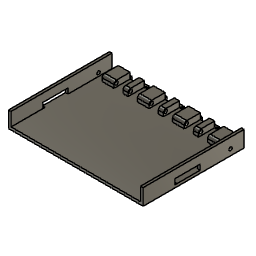
NEW+Key+Housing (Autodesk Fusion 360 design; units mm, degrees)
Autodesk Fusion 360 part; units mm, degrees
note: some values were not read from the file. Set by a fixed rule: which sketch regions a step uses.
sketch "Base" plane through (0, 0, 0) normal (0, 0, 1) x (1, 0, 0)
  line L0 (0, 0) -> (101.6, 0)
  line L1 (101.6, 0) -> (101.6, 76.2)
  line L2 (0, 0) -> (0, 76.2)
  line L3 (0, 76.2) -> (0, 78.74)
  line L4 (0, 78.74) -> (101.6, 78.74)
  line L5 (101.6, 78.74) -> (101.6, 76.2)
  dimension "d1" = 101.6
  dimension "d2" = 76.2
  dimension "d3" = 76.2
  dimension "d24" = 2.54
  dimension "d25" = 101.6
  constraint coincident L0.start L2.start
  constraint horizontal L0
  constraint perpendicular L0 L1
  constraint perpendicular L0 L2
  constraint perpendicular L3 L4
  constraint vertical L5
  measures "d1" distance of L0.start L0.end
  measures "d2" distance of L0.end L1.end
  measures "d3" distance of L0.start L2.end
  measures "d24" distance of L2.end L3.end
  measures "d25" distance of L3.end L4.end
extrude "Extrude1" add sketch "Base" along normal blind 2.032
sketch "back fins" plane through (0, 0, 2.032) normal (0, 0, 1) x (-1, 0, 0)
  line L0 (0, 0) -> (-101.6, 0)
  line L1 (-101.6, 0) -> (-101.6, -76.2)
  line L2 (-101.6, -76.2) -> (-101.6, -78.74)
  line L3 (0, -78.74) -> (0, 0)
  line L4 (0, -78.74) -> (0, -76.2)
  line L5 (0, -76.2) -> (-5.969, -76.2)
  line L6 (-16.129, -76.2) -> (-5.969, -76.2)
  line L7 (0, -78.74) -> (0, -76.2)
  line L8 (-5.969, -76.2) -> (0, -76.2)
  line L9 (-16.129, -76.2) -> (-21.209, -76.2)
  line L10 (-27.432, -76.2) -> (-21.209, -76.2)
  line L11 (-27.432, -76.2) -> (-32.512, -76.2)
  line L12 (-32.512, -76.2) -> (-42.672, -76.2)
  line L13 (-42.672, -76.2) -> (-47.752, -76.2)
  line L14 (-53.975, -76.2) -> (-59.055, -76.2)
  line L15 (-69.215, -76.2) -> (-59.055, -76.2)
  line L16 (-47.752, -76.2) -> (-53.975, -76.2)
  line L17 (-69.215, -76.2) -> (-74.295, -76.2)
  line L18 (-101.6, -78.74) -> (-101.6, -76.2)
  line L19 (-11.049, -76.2) -> (-11.049, -78.74)
  line L20 (-24.3205, -76.2) -> (-24.3205, -78.74)
  line L21 (-37.592, -76.2) -> (-37.592, -78.74)
  line L22 (-50.8635, -76.2) -> (-50.8635, -78.74)
  line L23 (-64.135, -76.2) -> (-64.135, -78.74)
  line L24 (-77.4065, -76.2) -> (-77.4065, -78.74)
  line L25 (-90.678, -76.2) -> (-90.678, -78.74)
  line L26 (-11.049, -78.74) -> (-7.6835, -78.74)
  line L27 (-11.049, -78.74) -> (-14.4145, -78.74)
  line L28 (-24.3205, -78.74) -> (-20.955, -78.74)
  line L29 (-24.3205, -78.74) -> (-27.686, -78.74)
  line L30 (-37.592, -78.74) -> (-40.9575, -78.74)
  line L31 (-50.8635, -78.74) -> (-47.498, -78.74)
  line L32 (-50.8635, -78.74) -> (-54.229, -78.74)
  line L33 (-64.135, -78.74) -> (-60.7695, -78.74)
  line L34 (-64.135, -78.74) -> (-67.5005, -78.74)
  line L35 (-77.4065, -78.74) -> (-80.772, -78.74)
  line L36 (-90.678, -78.74) -> (-87.3125, -78.74)
  line L37 (-90.678, -78.74) -> (-94.0435, -78.74)
  line L38 (-37.592, -78.74) -> (-34.2265, -78.74)
  line L39 (-74.295, -76.2) -> (-101.6, -76.2)
  line L40 (-7.6835, -78.74) -> (-7.6835, -77.47)
  line L41 (-7.6835, -77.47) -> (-8.9535, -77.47)
  line L42 (-8.9535, -77.47) -> (-8.9535, -76.2)
  line L43 (-14.4145, -78.74) -> (-14.4145, -77.47)
  line L44 (-14.4145, -77.47) -> (-13.1445, -77.47)
  line L45 (-13.1445, -77.47) -> (-13.1445, -76.2)
  line L46 (-20.955, -78.74) -> (-20.955, -77.47)
  line L47 (-20.955, -77.47) -> (-22.225, -77.47)
  line L48 (-22.225, -77.47) -> (-22.225, -76.2)
  line L49 (-27.686, -78.74) -> (-27.686, -77.47)
  line L50 (-27.686, -77.47) -> (-26.416, -77.47)
  line L51 (-26.416, -77.47) -> (-26.416, -76.2)
  line L52 (-34.2265, -78.74) -> (-34.2265, -77.47)
  line L53 (-34.2265, -77.47) -> (-35.4965, -77.47)
  line L54 (-35.4965, -77.47) -> (-35.4965, -76.2)
  line L55 (-40.9575, -78.74) -> (-40.9575, -77.47)
  line L56 (-40.9575, -77.47) -> (-39.6875, -77.47)
  line L57 (-39.6875, -77.47) -> (-39.6875, -76.2)
  line L58 (-47.498, -78.74) -> (-47.498, -77.47)
  line L59 (-47.498, -77.47) -> (-48.768, -77.47)
  line L60 (-48.768, -77.47) -> (-48.768, -76.2)
  line L61 (-54.229, -78.74) -> (-54.229, -77.47)
  line L62 (-54.229, -77.47) -> (-52.959, -77.47)
  line L63 (-52.959, -77.47) -> (-52.959, -76.2)
  line L64 (-60.7695, -78.74) -> (-60.7695, -77.47)
  line L65 (-67.5005, -78.74) -> (-67.5005, -77.47)
  line L66 (-60.7695, -77.47) -> (-62.0395, -77.47)
  line L67 (-67.5005, -77.47) -> (-66.2305, -77.47)
  line L68 (-62.0395, -77.47) -> (-62.0395, -76.2)
  line L69 (-66.2305, -77.47) -> (-66.2305, -76.2)
  line L70 (-80.772, -78.74) -> (-80.772, -77.47)
  line L71 (-22.4155, -76.2) -> (-26.2255, -76.2)
  line L72 (-80.772, -77.47) -> (-79.502, -77.47)
  line L73 (-79.502, -77.47) -> (-79.502, -76.2)
  line L74 (-77.4065, -78.74) -> (-74.0283, -78.74)
  line L75 (-74.0283, -78.74) -> (-74.0283, -77.47)
  line L76 (-74.0283, -77.47) -> (-75.2983, -77.47)
  line L77 (-75.2983, -77.47) -> (-75.2983, -76.2)
  line L78 (-87.3125, -78.74) -> (-87.3125, -77.47)
  line L79 (-87.3125, -77.47) -> (-88.5825, -77.47)
  line L80 (-88.5825, -77.47) -> (-88.5825, -76.2)
  line L81 (-94.0435, -78.74) -> (-94.0435, -77.47)
  line L82 (-94.0435, -77.47) -> (-92.7735, -77.47)
  line L83 (-92.7735, -77.47) -> (-92.7735, -76.2)
  line L84 (0, -76.2) -> (0, -78.74)
  line L85 (0, -78.74) -> (-7.6835, -78.74)
  line L86 (-14.4145, -78.74) -> (-20.955, -78.74)
  line L87 (-27.686, -78.74) -> (-34.2265, -78.74)
  line L88 (-40.9575, -78.74) -> (-47.498, -78.74)
  line L89 (-54.229, -78.74) -> (-60.7695, -78.74)
  line L90 (-67.5005, -78.74) -> (-74.0283, -78.74)
  line L91 (-80.772, -78.74) -> (-87.3125, -78.74)
  line L92 (-94.0435, -78.74) -> (-101.6, -78.74)
  dimension "d27" = 5.969
  dimension "d118" = 3.3655
  dimension "d119" = 3.3655
  dimension "d120" = 3.3655
  dimension "d121" = 3.3655
  dimension "d123" = 3.3655
  dimension "d124" = 3.3655
  dimension "d125" = 3.3655
  dimension "d126" = 3.3655
  dimension "d127" = 3.3655
  dimension "d129" = 3.3655
  dimension "d130" = 3.3655
  dimension "d131" = 3.3655
  dimension "d132" = 3.3655
  dimension "d133" = 1.27
  dimension "d134" = 1.27
  dimension "d135" = 1.27
  dimension "d136" = 1.27
  dimension "d137" = 1.27
  dimension "d138" = 1.27
  dimension "d139" = 1.27
  dimension "d140" = 1.27
  dimension "d141" = 1.27
  dimension "d142" = 1.27
  dimension "d143" = 1.27
  dimension "d144" = 1.27
  dimension "d145" = 1.27
  dimension "d146" = 1.27
  dimension "d147" = 1.27
  dimension "d148" = 1.27
  dimension "d149" = 1.27
  dimension "d150" = 1.27
  dimension "d151" = 1.27
  dimension "d152" = 1.27
  dimension "d153" = 1.27
  dimension "d156" = 1.27
  dimension "d157" = 3.81
  dimension "d159" = 1.27
  dimension "d161" = 3.3782
  dimension "d162" = 1.27
  dimension "d163" = 1.27
  dimension "d164" = 1.27
  dimension "d165" = 1.27
  dimension "d166" = 1.27
  dimension "d167" = 1.27
  constraint coincident L3.start L4.start
  constraint coincident L3 L4.end
  constraint perpendicular L4 L5
  constraint coincident L2.end L18.start
  constraint coincident L1.end L2.start
  constraint midpoint L6 L19.start
  constraint midpoint L10 L20.start
  constraint midpoint L12 L21.start
  constraint midpoint L16 L22.start
  constraint midpoint L15 L23.start
  constraint perpendicular L19 L26
  constraint perpendicular L19 L27
  constraint perpendicular L20 L28
  constraint perpendicular L20 L29
  constraint perpendicular L21 L30
  constraint perpendicular L22 L31
  constraint perpendicular L22 L32
  constraint perpendicular L23 L33
  constraint perpendicular L23 L34
  constraint perpendicular L24 L35
  constraint perpendicular L25 L36
  constraint perpendicular L25 L37
  constraint perpendicular L21 L38
  constraint perpendicular L26 L40
  constraint perpendicular L40 L41
  constraint coincident L6 L42.end
  constraint perpendicular L6 L42
  constraint perpendicular L27 L43
  constraint perpendicular L43 L44
  constraint coincident L6 L45.end
  constraint perpendicular L6 L45
  constraint perpendicular L28 L46
  constraint perpendicular L46 L47
  constraint coincident L10 L48.end
  constraint perpendicular L10 L48
  constraint perpendicular L29 L49
  constraint perpendicular L49 L50
  constraint coincident L10 L51.end
  constraint perpendicular L10 L51
  constraint perpendicular L38 L52
  constraint perpendicular L52 L53
  constraint coincident L12 L54.end
  constraint perpendicular L12 L54
  constraint perpendicular L30 L55
  constraint perpendicular L55 L56
  constraint coincident L12 L57.end
  constraint perpendicular L12 L57
  constraint perpendicular L31 L58
  constraint perpendicular L58 L59
  constraint coincident L16 L60.end
  constraint perpendicular L16 L60
  constraint perpendicular L32 L61
  constraint perpendicular L61 L62
  constraint perpendicular L16 L63
  constraint perpendicular L33 L64
  constraint perpendicular L34 L65
  constraint perpendicular L64 L66
  constraint perpendicular L65 L67
  constraint coincident L15 L68.end
  constraint perpendicular L15 L68
  constraint coincident L15 L69.end
  constraint perpendicular L15 L69
  constraint perpendicular L35 L70
  constraint horizontal L71
  constraint perpendicular L70 L72
  constraint coincident L39 L73.end
  constraint perpendicular L39 L73
  constraint perpendicular L24 L74
  constraint perpendicular L74 L75
  constraint perpendicular L75 L76
  constraint coincident L39 L77.end
  constraint perpendicular L39 L77
  constraint perpendicular L36 L78
  constraint perpendicular L78 L79
  constraint coincident L39 L80.end
  constraint perpendicular L39 L80
  constraint perpendicular L37 L81
  constraint perpendicular L81 L82
  constraint coincident L39 L83.end
  constraint perpendicular L39 L83
  constraint perpendicular L40 L85
  constraint perpendicular L46 L86
  constraint perpendicular L52 L87
  constraint perpendicular L58 L88
  constraint perpendicular L64 L89
  constraint perpendicular L75 L90
  constraint perpendicular L78 L91
  constraint parallel L37 L92
  measures "d27" distance of L4.end L5.end
  measures "d118" distance of L19.end L26.end
  measures "d119" distance of L19.end L27.end
  measures "d120" distance of L20.end L28.end
  measures "d121" distance of L20.end L29.end
  measures "d123" distance of L21.end L30.end
  measures "d124" distance of L22.end L31.end
  measures "d125" distance of L22.end L32.end
  measures "d126" distance of L23.end L33.end
  measures "d127" distance of L23.end L34.end
  measures "d129" distance of L24.end L35.end
  measures "d130" distance of L25.end L36.end
  measures "d131" distance of L25.end L37.end
  measures "d132" distance of L21.end L38.end
  measures "d133" distance of L26.end L40.end
  measures "d134" distance of L40.end L41.end
  measures "d135" distance of L27.end L43.end
  measures "d136" distance of L43.end L44.end
  measures "d137" distance of L28.end L46.end
  measures "d138" distance of L46.end L47.end
  measures "d139" distance of L29.end L49.end
  measures "d140" distance of L49.end L50.end
  measures "d141" distance of L38.end L52.end
  measures "d142" distance of L52.end L53.end
  measures "d143" distance of L30.end L55.end
  measures "d144" distance of L55.end L56.end
  measures "d145" distance of L31.end L58.end
  measures "d146" distance of L58.end L59.end
  measures "d147" distance of L32.end L61.end
  measures "d148" distance of L61.end L62.end
  measures "d149" distance of L62.end L63.end
  measures "d150" distance of L33.end L64.end
  measures "d151" distance of L34.end L65.end
  measures "d152" distance of L64.end L66.end
  measures "d153" distance of L65.end L67.end
  measures "d156" distance of L35.end L70.end
  measures "d157" distance of L71.end L71.start
  measures "d159" distance of L70.end L72.end
  measures "d161" distance of L24.end L74.end
  measures "d162" distance of L74.end L75.end
  measures "d163" distance of L75.end L76.end
  measures "d164" distance of L36.end L78.end
  measures "d165" distance of L78.end L79.end
  measures "d166" distance of L37.end L81.end
  measures "d167" distance of L81.end L82.end
extrude "Extrude3" cut sketch "back fins" against normal blind 2.54 contours L3 L4 L5 L6 L7 L8 L40 L41 L42 L84 L85 | L2 L18 L39 L81 L82 L83 L92 | L39 L70 L72 L73 L78 L79 L80 L91 | L6 L9 L10 L43 L44 L45 L46 L47 L48 L86 | L15 L17 L39 L65 L67 L69 L75 L76 L77 L90 | L10 L11 L12 L49 L50 L51 L52 L53 L54 L87 | L12 L13 L16 L55 L56 L57 L58 L59 L60 L88 | L14 L15 L16 L61 L62 L63 L64 L66 L68 L89
sketch "axel fins" plane through (0, 0, 2.032) normal (0, 0, 1) x (-1, 0, 0)
  line L0 (-27.686, -78.74) -> (-20.955, -78.74)
  line L1 (-11.049, -78.74) -> (-11.049, -77.724)
  line L2 (-24.3205, -78.74) -> (-24.3205, -77.724)
  line L3 (-37.592, -78.74) -> (-37.592, -77.724)
  line L4 (-50.8635, -78.74) -> (-50.8635, -77.978)
  line L5 (-64.135, -78.74) -> (-64.135, -77.978)
  line L6 (-77.4065, -78.74) -> (-77.4065, -77.724)
  line L7 (-90.678, -78.74) -> (-90.678, -77.978)
  line L8 (-6.604, -76.2) -> (-15.494, -76.2)
  line L9 (-15.494, -76.2) -> (-15.494, -66.04)
  line L10 (-6.604, -66.04) -> (-6.604, -76.2)
  line L11 (-11.049, -76.2) -> (-11.049, -66.04)
  line L12 (-33.147, -76.2) -> (-42.037, -76.2)
  line L13 (-33.147, -60.96) -> (-33.147, -76.2)
  line L14 (-37.592, -76.2) -> (-37.592, -60.96)
  line L15 (-42.037, -60.96) -> (-33.147, -60.96)
  line L16 (-42.037, -76.2) -> (-42.037, -60.96)
  line L17 (-59.69, -76.2) -> (-68.58, -76.2)
  line L18 (-59.69, -60.96) -> (-59.69, -76.2)
  line L19 (-64.135, -76.2) -> (-64.135, -60.96)
  line L20 (-68.58, -60.96) -> (-59.69, -60.96)
  line L21 (-68.58, -76.2) -> (-68.58, -60.96)
  line L22 (-86.233, -76.2) -> (-95.123, -76.2)
  line L23 (-86.233, -60.96) -> (-86.233, -76.2)
  line L24 (-90.678, -76.2) -> (-90.678, -60.96)
  line L25 (-95.123, -60.96) -> (-86.233, -60.96)
  line L26 (-95.123, -76.2) -> (-95.123, -60.96)
  line L27 (-22.4155, -76.2) -> (-26.2255, -76.2)
  line L28 (-26.2255, -76.2) -> (-26.2255, -60.96)
  line L29 (-26.2255, -60.96) -> (-22.4155, -60.96)
  line L30 (-22.4155, -60.96) -> (-22.4155, -76.2)
  line L31 (-24.3205, -76.2) -> (-24.3205, -60.96)
  line L32 (-6.604, -76.2) -> (-15.494, -76.2)
  line L33 (-6.604, -66.04) -> (-6.604, -76.2)
  line L34 (-11.049, -76.2) -> (-11.049, -66.04)
  line L35 (-15.494, -76.2) -> (-15.494, -66.04)
  line L36 (-6.604, -76.2) -> (-15.494, -76.2)
  line L37 (-6.604, -60.96) -> (-6.604, -76.2)
  line L38 (-11.049, -76.2) -> (-11.049, -60.96)
  line L39 (-15.494, -60.96) -> (-6.604, -60.96)
  line L40 (-15.494, -76.2) -> (-15.494, -60.96)
  line L41 (-48.9585, -76.2) -> (-52.7685, -76.2)
  line L42 (-48.9585, -60.96) -> (-48.9585, -76.2)
  line L43 (-50.8635, -76.2) -> (-50.8635, -60.96)
  line L44 (-52.7685, -76.2) -> (-52.7685, -60.96)
  line L45 (-52.7685, -60.96) -> (-48.9585, -60.96)
  line L46 (-75.5015, -76.2) -> (-79.3115, -76.2)
  line L47 (-75.5015, -60.96) -> (-75.5015, -76.2)
  line L48 (-77.4065, -76.2) -> (-77.4065, -60.96)
  line L49 (-79.3115, -76.2) -> (-79.3115, -60.96)
  line L50 (-79.3115, -60.96) -> (-75.5015, -60.96)
  line L51 (-74.0283, -78.74) -> (-74.0283, -77.47)
  line L52 (-74.0283, -77.47) -> (-75.2983, -77.47)
  line L53 (-75.2983, -77.47) -> (-75.2983, -76.2)
  line L54 (-101.6, -76.2) -> (-92.7735, -76.2)
  line L55 (-7.6835, -78.74) -> (-7.6835, -77.47)
  line L56 (-7.6835, -77.47) -> (-8.9535, -77.47)
  line L57 (-8.9535, -77.47) -> (-8.9535, -76.2)
  line L58 (-21.209, -76.2) -> (-13.1445, -76.2)
  line L59 (-13.1445, -76.2) -> (-13.1445, -77.47)
  line L60 (-13.1445, -77.47) -> (-14.4145, -77.47)
  line L61 (-14.4145, -77.47) -> (-14.4145, -78.74)
  line L62 (-67.5005, -77.47) -> (-67.5005, -78.74)
  line L63 (-67.5005, -78.74) -> (-60.7695, -78.74)
  line L64 (-60.7695, -78.74) -> (-60.7695, -77.47)
  line L65 (-60.7695, -77.47) -> (-62.0395, -77.47)
  line L66 (-62.0395, -77.47) -> (-62.0395, -76.2)
  line L67 (-62.0395, -76.2) -> (-59.055, -76.2)
  line L68 (-66.2305, -76.2) -> (-66.2305, -77.47)
  line L69 (-66.2305, -77.47) -> (-67.5005, -77.47)
  line L70 (-54.229, -77.47) -> (-54.229, -78.74)
  line L71 (-54.229, -78.74) -> (-47.498, -78.74)
  line L72 (-47.498, -78.74) -> (-47.498, -77.47)
  line L73 (-47.498, -77.47) -> (-48.768, -77.47)
  line L74 (-48.768, -77.47) -> (-48.768, -76.2)
  line L75 (-59.055, -76.2) -> (-52.959, -76.2)
  line L76 (-52.959, -76.2) -> (-52.959, -77.47)
  line L77 (-52.959, -77.47) -> (-54.229, -77.47)
  line L78 (-92.7735, -76.2) -> (-92.7735, -77.47)
  line L79 (-92.7735, -77.47) -> (-94.0435, -77.47)
  line L80 (-94.0435, -77.47) -> (-94.0435, -78.74)
  line L81 (-94.0435, -78.74) -> (-87.3125, -78.74)
  line L82 (-40.9575, -77.47) -> (-40.9575, -78.74)
  line L83 (-40.9575, -78.74) -> (-34.2265, -78.74)
  line L84 (-34.2265, -78.74) -> (-34.2265, -77.47)
  line L85 (-34.2265, -77.47) -> (-35.4965, -77.47)
  line L86 (-35.4965, -77.47) -> (-35.4965, -76.2)
  line L87 (-48.768, -76.2) -> (-39.6875, -76.2)
  line L88 (-39.6875, -76.2) -> (-39.6875, -77.47)
  line L89 (-39.6875, -77.47) -> (-40.9575, -77.47)
  line L90 (-35.4965, -76.2) -> (-27.432, -76.2)
  line L91 (-27.432, -76.2) -> (-26.416, -76.2)
  line L92 (-26.416, -76.2) -> (-26.416, -77.47)
  line L93 (-26.416, -77.47) -> (-27.686, -77.47)
  line L94 (-27.686, -77.47) -> (-27.686, -78.74)
  line L95 (-20.955, -78.74) -> (-20.955, -77.47)
  line L96 (-20.955, -77.47) -> (-22.225, -77.47)
  line L97 (-22.225, -77.47) -> (-22.225, -76.2)
  line L98 (-22.225, -76.2) -> (-21.209, -76.2)
  line L99 (-14.4145, -78.74) -> (-7.6835, -78.74)
  line L100 (-8.9535, -76.2) -> (0, -76.2)
  line L101 (0, -76.2) -> (0, 0)
  line L102 (0, 0) -> (-101.6, 0)
  line L103 (-101.6, 0) -> (-101.6, -76.2)
  line L104 (-87.3125, -78.74) -> (-87.3125, -77.47)
  line L105 (-87.3125, -77.47) -> (-88.5825, -77.47)
  line L106 (-88.5825, -77.47) -> (-88.5825, -76.2)
  line L107 (-88.5825, -76.2) -> (-79.502, -76.2)
  line L108 (-79.502, -76.2) -> (-79.502, -77.47)
  line L109 (-79.502, -77.47) -> (-80.772, -77.47)
  line L110 (-80.772, -77.47) -> (-80.772, -78.74)
  line L111 (-80.772, -78.74) -> (-74.0283, -78.74)
  line L112 (-75.2983, -76.2) -> (-74.295, -76.2)
  line L113 (-74.295, -76.2) -> (-69.215, -76.2)
  line L114 (-69.215, -76.2) -> (-66.2305, -76.2)
  dimension "d70" = 8.89
  dimension "d71" = 8.89
  dimension "d72" = 8.89
  dimension "d73" = 8.89
  dimension "d74" = 3.81
  dimension "d75" = 8.89
  dimension "d76" = 8.89
  dimension "d77" = 3.81
  dimension "d78" = 3.81
  dimension "d84" = 15.24
  dimension "d85" = 15.24
  dimension "d86" = 15.24
  dimension "d87" = 15.24
  dimension "d88" = 15.24
  dimension "d89" = 15.24
  dimension "d90" = 15.24
  constraint midpoint L0 L5.start
  constraint perpendicular L0 L5
  constraint horizontal L8
  constraint vertical L9
  constraint vertical L10
  constraint midpoint L8 L11.start
  constraint horizontal L12
  constraint vertical L16
  constraint horizontal L15
  constraint vertical L13
  constraint midpoint L14.start L12
  constraint midpoint L14.end L15
  constraint horizontal L17
  constraint vertical L21
  constraint horizontal L20
  constraint vertical L18
  constraint midpoint L19.start L17
  constraint midpoint L19.end L20
  constraint horizontal L22
  constraint vertical L26
  constraint horizontal L25
  constraint vertical L23
  constraint midpoint L24.start L22
  constraint midpoint L24.end L25
  constraint collinear L1 L11
  constraint collinear L3 L14
  constraint collinear L5 L19
  constraint collinear L7 L24
  constraint horizontal L27
  constraint vertical L28
  constraint horizontal L29
  constraint vertical L30
  constraint midpoint L27 L31.start
  constraint midpoint L29 L31.end
  constraint collinear L2 L31
  constraint horizontal L32
  constraint vertical L35
  constraint vertical L33
  constraint midpoint L11.start L32
  constraint horizontal L36
  constraint vertical L40
  constraint horizontal L39
  constraint vertical L37
  constraint midpoint L11.start L36
  constraint midpoint L38.end L39
  constraint horizontal L41
  constraint vertical L44
  constraint horizontal L45
  constraint vertical L42
  constraint midpoint L43.start L41
  constraint midpoint L43.end L45
  constraint horizontal L46
  constraint vertical L49
  constraint horizontal L50
  constraint vertical L47
  constraint midpoint L48.start L46
  constraint midpoint L48.end L50
  constraint collinear L6 L48
  constraint collinear L4 L43
  measures "d70" distance of L8.start L8.end
  measures "d71" distance of L12.end L12.start
  measures "d72" distance of L17.end L17.start
  measures "d73" distance of L22.end L22.start
  measures "d74" distance of L27.start L27.end
  measures "d75" distance of L8.end L8.start
  measures "d76" distance of L8.end L8.start
  measures "d77" distance of L41.end L41.start
  measures "d78" distance of L46.end L46.start
  measures "d84" distance of L8.start L37.start
  measures "d85" distance of L27.start L29.end
  measures "d86" distance of L12.start L13.start
  measures "d87" distance of L42.start L41.start
  measures "d88" distance of L17.start L18.start
  measures "d89" distance of L47.start L46.start
  measures "d90" distance of L22.start L23.start
extrude "Extrude4" add sketch "axel fins" along normal blind 4.445 contours L12 L13 L14 L15 L90 | L8 L9 L11 L32 L34 L35 L36 L38 L39 L40 L58 | L12 L14 L15 L16 L87 | L8 L10 L11 L32 L33 L34 L36 L37 L38 L39 L100 | L22 L24 L25 L26 L54 | L22 L23 L24 L25 L107 | L17 L18 L19 L20 L67 | L17 L19 L20 L21 L114 | L27 L29 L30 L31 | L27 L28 L29 L31 | L41 L42 L43 L45 | L41 L43 L44 L45 | L46 L47 L48 L50 | L46 L48 L49 L50
sketch "walls" plane through (0, 0, 2.032) normal (0, 0, 1) x (-1, 0, 0)
  line L0 (-94.0435, -78.74) -> (-87.3125, -78.74)
  line L1 (-101.6, 0) -> (-99.695, 0)
  line L2 (-99.695, 0) -> (-99.694, -76.2)
  line L3 (0, 0) -> (-1.905, 0)
  line L4 (-1.905, -76.2) -> (0, -76.2)
  line L5 (0, -76.2) -> (0, 0)
  line L6 (-1.905, 0) -> (-1.905, -76.2)
  line L7 (-6.604, -60.96) -> (-6.604, -76.2)
  line L8 (-6.604, -76.2) -> (0, -76.2)
  line L9 (0, -76.2) -> (0, 0)
  line L10 (0, 0) -> (-101.6, 0)
  line L11 (-101.6, 0) -> (-101.6, -76.2)
  line L12 (-101.6, -76.2) -> (-92.7735, -76.2)
  line L13 (-92.7735, -76.2) -> (-92.7735, -77.47)
  line L14 (-92.7735, -77.47) -> (-94.0435, -77.47)
  line L15 (-94.0435, -77.47) -> (-94.0435, -78.74)
  line L16 (-87.3125, -78.74) -> (-87.3125, -77.47)
  line L17 (-87.3125, -77.47) -> (-88.5825, -77.47)
  line L18 (-88.5825, -77.47) -> (-88.5825, -76.2)
  line L19 (-88.5825, -76.2) -> (-86.233, -76.2)
  line L20 (-86.233, -76.2) -> (-95.123, -76.2)
  line L21 (-95.123, -76.2) -> (-95.123, -60.96)
  line L22 (-95.123, -60.96) -> (-86.233, -60.96)
  line L23 (-86.233, -60.96) -> (-86.233, -76.2)
  line L24 (-86.233, -76.2) -> (-79.502, -76.2)
  line L25 (-79.502, -76.2) -> (-79.502, -77.47)
  line L26 (-79.502, -77.47) -> (-80.772, -77.47)
  line L27 (-80.772, -77.47) -> (-80.772, -78.74)
  line L28 (-80.772, -78.74) -> (-74.0283, -78.74)
  line L29 (-74.0283, -78.74) -> (-74.0283, -77.47)
  line L30 (-74.0283, -77.47) -> (-75.2983, -77.47)
  line L31 (-75.2983, -77.47) -> (-75.2983, -76.2)
  line L32 (-75.2983, -76.2) -> (-74.295, -76.2)
  line L33 (-74.295, -76.2) -> (-69.215, -76.2)
  line L34 (-69.215, -76.2) -> (-68.58, -76.2)
  line L35 (-68.58, -76.2) -> (-68.58, -60.96)
  line L36 (-68.58, -60.96) -> (-59.69, -60.96)
  line L37 (-59.69, -60.96) -> (-59.69, -76.2)
  line L38 (-59.69, -76.2) -> (-66.2305, -76.2)
  line L39 (-66.2305, -76.2) -> (-66.2305, -77.47)
  line L40 (-66.2305, -77.47) -> (-67.5005, -77.47)
  line L41 (-67.5005, -77.47) -> (-67.5005, -78.74)
  line L42 (-67.5005, -78.74) -> (-60.7695, -78.74)
  line L43 (-60.7695, -78.74) -> (-60.7695, -77.47)
  line L44 (-60.7695, -77.47) -> (-62.0395, -77.47)
  line L45 (-62.0395, -77.47) -> (-62.0395, -76.2)
  line L46 (-62.0395, -76.2) -> (-59.055, -76.2)
  line L47 (-59.055, -76.2) -> (-52.959, -76.2)
  line L48 (-52.959, -76.2) -> (-52.959, -77.47)
  line L49 (-52.959, -77.47) -> (-54.229, -77.47)
  line L50 (-54.229, -77.47) -> (-54.229, -78.74)
  line L51 (-54.229, -78.74) -> (-47.498, -78.74)
  line L52 (-47.498, -78.74) -> (-47.498, -77.47)
  line L53 (-47.498, -77.47) -> (-48.768, -77.47)
  line L54 (-48.768, -77.47) -> (-48.768, -76.2)
  line L55 (-48.768, -76.2) -> (-39.6875, -76.2)
  line L56 (-39.6875, -76.2) -> (-39.6875, -77.47)
  line L57 (-39.6875, -77.47) -> (-40.9575, -77.47)
  line L58 (-40.9575, -77.47) -> (-40.9575, -78.74)
  line L59 (-40.9575, -78.74) -> (-34.2265, -78.74)
  line L60 (-34.2265, -78.74) -> (-34.2265, -77.47)
  line L61 (-34.2265, -77.47) -> (-35.4965, -77.47)
  line L62 (-35.4965, -77.47) -> (-35.4965, -76.2)
  line L63 (-35.4965, -76.2) -> (-27.432, -76.2)
  line L64 (-27.432, -76.2) -> (-26.416, -76.2)
  line L65 (-26.416, -76.2) -> (-26.416, -77.47)
  line L66 (-26.416, -77.47) -> (-27.686, -77.47)
  line L67 (-27.686, -77.47) -> (-27.686, -78.74)
  line L68 (-27.686, -78.74) -> (-20.955, -78.74)
  line L69 (-20.955, -78.74) -> (-20.955, -77.47)
  line L70 (-20.955, -77.47) -> (-22.225, -77.47)
  line L71 (-22.225, -77.47) -> (-22.225, -76.2)
  line L72 (-22.225, -76.2) -> (-21.209, -76.2)
  line L73 (-21.209, -76.2) -> (-15.494, -76.2)
  line L74 (-15.494, -76.2) -> (-15.494, -60.96)
  line L75 (-15.494, -60.96) -> (-6.604, -60.96)
  line L76 (-52.7685, -60.96) -> (-48.9585, -60.96)
  line L77 (-48.9585, -60.96) -> (-48.9585, -76.2)
  line L78 (-48.9585, -76.2) -> (-52.7685, -76.2)
  line L79 (-52.7685, -76.2) -> (-52.7685, -60.96)
  line L80 (-79.3115, -60.96) -> (-75.5015, -60.96)
  line L81 (-75.5015, -60.96) -> (-75.5015, -76.2)
  line L82 (-75.5015, -76.2) -> (-79.3115, -76.2)
  line L83 (-79.3115, -76.2) -> (-79.3115, -60.96)
  line L84 (-22.4155, -60.96) -> (-22.4155, -76.2)
  line L85 (-22.4155, -76.2) -> (-26.2255, -76.2)
  line L86 (-26.2255, -76.2) -> (-26.2255, -60.96)
  line L87 (-26.2255, -60.96) -> (-22.4155, -60.96)
  line L88 (-42.037, -76.2) -> (-42.037, -60.96)
  line L89 (-42.037, -60.96) -> (-33.147, -60.96)
  line L90 (-33.147, -60.96) -> (-33.147, -76.2)
  line L91 (-33.147, -76.2) -> (-42.037, -76.2)
  line L92 (-99.694, -76.2) -> (-101.6, -76.2)
  line L93 (-101.6, 0) -> (-101.6, -76.2)
  dimension "d81" = 1.905
  dimension "d97" = 1.905
  constraint coincident L3.start L5.end
  constraint coincident L11.end L12.start
  constraint parallel L11 L93
  measures "d81" distance of L1.start L1.end
  measures "d97" distance of L3.start L3.end
extrude "Extrude5" add sketch "walls" along normal blind 10.16 contours L1 L2 L10 L11 L12 L92 L93 | L3 L4 L5 L6 L8 L9 L10
sketch "Axis hole" plane through (101.6, 0, 0) normal (1, 0, 0) x (0, 1, 0)
  line L0 (0, 0) -> (76.2, 0)
  line L1 (0, 12.192) -> (0, 0)
  line L2 (76.2, 12.192) -> (66.04, 12.192)
  line L3 (76.2, 0) -> (66.04, 0)
  line L4 (76.2, 1.9774) -> (66.04, 1.9774)
  line L5 (66.04, 1.9774) -> (66.04, 4.5174)
  circle A0 centre (66.04, 4.5174) radius 1.27
  line L6 (76.2, 0) -> (76.2, 2.032)
  line L7 (76.2, 2.032) -> (76.2, 12.192)
  line L8 (76.2, 12.192) -> (0, 12.192)
  dimension "d91" = 10.16
  dimension "d93" = 2.54
  dimension "d94" = 2.54
  constraint coincident L0.end L3.start
  constraint coincident L0 L3.end
  constraint perpendicular L4 L5
  constraint coincident L5.end A0.centre
  measures "d91" distance of L2.start L2.end
  measures "d93" distance of L4.end L5.end
  measures "d94" diameter of A0
extrude "Extrude6" cut sketch "Axis hole" against normal blind 104.14 contours A0
sketch "Sketch8" plane through (95.123, 0, 0) normal (1, 0, 0) x (0, 1, 0)
  circle A0 centre (66.04, 4.5174) radius 1.27
  line L0 (76.2, 2.032) -> (76.2, 6.477)
  line L1 (76.2, 6.477) -> (60.96, 6.477)
  line L2 (60.96, 6.477) -> (60.96, 2.032)
  line L3 (66.04, 6.477) -> (60.96, 6.477)
  line L4 (64.0804, 2.032) -> (60.96, 2.032)
  line L5 (60.96, 6.477) -> (60.96, 2.032)
  line L6 (64.0804, 4.5174) -> (64.0804, 2.032)
  arc A1 (66.04, 6.477) -> (64.0804, 4.5174) centre (66.04, 4.5174) ccw
  line L7 (60.96, 2.032) -> (76.2, 2.032)
  constraint concentric A0 A1
  constraint tangent L1 A1
  constraint coincident L1 L3.start
  constraint coincident L1.end L2.start
  constraint coincident L2.end L4.end
  constraint perpendicular L2 L4
  constraint tangent L6 A1
extrude "Extrude7" cut sketch "Sketch8" against normal blind 91.44 contours L1 L2 L3 L4 L5 L6 A1 L7
sketch "Sketch9" plane through (0, 0, 2.032) normal (0, 0, 1) x (-1, 0, 0)
  line L0 (-94.0435, -78.74) -> (-87.3125, -78.74)
  line L1 (-11.049, -78.74) -> (-11.049, -78.0889)
  circle A0 centre (-11.049, -22.8439) radius 3.81
  line L2 (-11.049, -22.8439) -> (-11.049, -58.928)
  line L3 (-11.049, -22.8439) -> (-11.049, -78.0889)
  line L4 (-37.592, -78.74) -> (-37.592, -23.495)
  line L5 (-64.135, -78.74) -> (-64.135, -23.495)
  line L6 (-90.678, -78.74) -> (-90.678, -23.495)
  circle A1 centre (-37.592, -23.495) radius 3.81
  circle A2 centre (-64.135, -23.495) radius 3.81
  circle A3 centre (-90.678, -23.495) radius 3.81
  line L7 (-6.604, -64.0804) -> (-6.604, -76.2)
  line L8 (-6.604, -76.2) -> (-1.905, -76.2)
  line L9 (-1.905, -76.2) -> (-1.905, 0)
  line L10 (-1.905, 0) -> (-99.695, 0)
  line L11 (-101.6, -76.2) -> (-92.7735, -76.2)
  line L12 (-92.7735, -76.2) -> (-92.7735, -77.47)
  line L13 (-92.7735, -77.47) -> (-94.0435, -77.47)
  line L14 (-94.0435, -77.47) -> (-94.0435, -78.74)
  line L15 (-87.3125, -78.74) -> (-87.3125, -77.47)
  line L16 (-87.3125, -77.47) -> (-88.5825, -77.47)
  line L17 (-88.5825, -77.47) -> (-88.5825, -76.2)
  line L18 (-88.5825, -76.2) -> (-86.233, -76.2)
  line L19 (-86.233, -76.2) -> (-95.123, -76.2)
  line L20 (-95.123, -76.2) -> (-95.123, -64.0804)
  line L21 (-95.123, -64.0804) -> (-86.233, -64.0804)
  line L22 (-86.233, -64.0804) -> (-86.233, -76.2)
  line L23 (-86.233, -76.2) -> (-79.502, -76.2)
  line L24 (-79.502, -76.2) -> (-79.502, -77.47)
  line L25 (-79.502, -77.47) -> (-80.772, -77.47)
  line L26 (-80.772, -77.47) -> (-80.772, -78.74)
  line L27 (-80.772, -78.74) -> (-74.0283, -78.74)
  line L28 (-74.0283, -78.74) -> (-74.0283, -77.47)
  line L29 (-74.0283, -77.47) -> (-75.2983, -77.47)
  line L30 (-75.2983, -77.47) -> (-75.2983, -76.2)
  line L31 (-75.2983, -76.2) -> (-74.295, -76.2)
  line L32 (-74.295, -76.2) -> (-69.215, -76.2)
  line L33 (-69.215, -76.2) -> (-68.58, -76.2)
  line L34 (-68.58, -76.2) -> (-68.58, -64.0804)
  line L35 (-68.58, -64.0804) -> (-59.69, -64.0804)
  line L36 (-59.69, -64.0804) -> (-59.69, -76.2)
  line L37 (-59.69, -76.2) -> (-66.2305, -76.2)
  line L38 (-66.2305, -76.2) -> (-66.2305, -77.47)
  line L39 (-66.2305, -77.47) -> (-67.5005, -77.47)
  line L40 (-67.5005, -77.47) -> (-67.5005, -78.74)
  line L41 (-67.5005, -78.74) -> (-60.7695, -78.74)
  line L42 (-60.7695, -78.74) -> (-60.7695, -77.47)
  line L43 (-60.7695, -77.47) -> (-62.0395, -77.47)
  line L44 (-62.0395, -77.47) -> (-62.0395, -76.2)
  line L45 (-62.0395, -76.2) -> (-59.055, -76.2)
  line L46 (-59.055, -76.2) -> (-52.959, -76.2)
  line L47 (-52.959, -76.2) -> (-52.959, -77.47)
  line L48 (-52.959, -77.47) -> (-54.229, -77.47)
  line L49 (-54.229, -77.47) -> (-54.229, -78.74)
  line L50 (-54.229, -78.74) -> (-47.498, -78.74)
  line L51 (-47.498, -78.74) -> (-47.498, -77.47)
  line L52 (-47.498, -77.47) -> (-48.768, -77.47)
  line L53 (-48.768, -77.47) -> (-48.768, -76.2)
  line L54 (-48.768, -76.2) -> (-39.6875, -76.2)
  line L55 (-39.6875, -76.2) -> (-39.6875, -77.47)
  line L56 (-39.6875, -77.47) -> (-40.9575, -77.47)
  line L57 (-40.9575, -77.47) -> (-40.9575, -78.74)
  line L58 (-40.9575, -78.74) -> (-34.2265, -78.74)
  line L59 (-34.2265, -78.74) -> (-34.2265, -77.47)
  line L60 (-34.2265, -77.47) -> (-35.4965, -77.47)
  line L61 (-35.4965, -77.47) -> (-35.4965, -76.2)
  line L62 (-35.4965, -76.2) -> (-27.432, -76.2)
  line L63 (-27.432, -76.2) -> (-26.416, -76.2)
  line L64 (-26.416, -76.2) -> (-26.416, -77.47)
  line L65 (-26.416, -77.47) -> (-27.686, -77.47)
  line L66 (-27.686, -77.47) -> (-27.686, -78.74)
  line L67 (-27.686, -78.74) -> (-20.955, -78.74)
  line L68 (-20.955, -78.74) -> (-20.955, -77.47)
  line L69 (-20.955, -77.47) -> (-22.225, -77.47)
  line L70 (-22.225, -77.47) -> (-22.225, -76.2)
  line L71 (-22.225, -76.2) -> (-21.209, -76.2)
  line L72 (-21.209, -76.2) -> (-15.494, -76.2)
  line L73 (-15.494, -76.2) -> (-15.494, -64.0804)
  line L74 (-15.494, -64.0804) -> (-6.604, -64.0804)
  line L75 (-75.5015, -64.0804) -> (-75.5015, -76.2)
  line L76 (-75.5015, -76.2) -> (-79.3115, -76.2)
  line L77 (-79.3115, -76.2) -> (-79.3115, -64.0804)
  line L78 (-79.3115, -64.0804) -> (-75.5015, -64.0804)
  line L79 (-22.4155, -64.0804) -> (-22.4155, -76.2)
  line L80 (-22.4155, -76.2) -> (-26.2255, -76.2)
  line L81 (-26.2255, -76.2) -> (-26.2255, -64.0804)
  line L82 (-26.2255, -64.0804) -> (-22.4155, -64.0804)
  line L83 (-48.9585, -64.0804) -> (-48.9585, -76.2)
  line L84 (-48.9585, -76.2) -> (-52.7685, -76.2)
  line L85 (-52.7685, -76.2) -> (-52.7685, -64.0804)
  line L86 (-52.7685, -64.0804) -> (-48.9585, -64.0804)
  line L87 (-33.147, -64.0804) -> (-33.147, -76.2)
  line L88 (-33.147, -76.2) -> (-42.037, -76.2)
  line L89 (-42.037, -76.2) -> (-42.037, -64.0804)
  line L90 (-42.037, -64.0804) -> (-33.147, -64.0804)
  line L91 (-99.695, 0) -> (-99.694, -76.2)
  line L92 (-99.694, -76.2) -> (-101.6, -76.2)
  dimension "d100" = 7.62
  dimension "d101" = 55.245
  dimension "d104" = 55.245
  dimension "d105" = 55.245
  dimension "d106" = 55.245
  dimension "d107" = 7.62
  dimension "d108" = 7.62
  dimension "d109" = 7.62
  constraint coincident A0.centre L2.start
  constraint collinear L1 L2
  constraint midpoint L0 L6.start
  constraint coincident L4.end A1.centre
  constraint coincident L5.end A2.centre
  constraint coincident L6.end A3.centre
  measures "d100" diameter of A0
  measures "d101" distance of L1.end A0.centre
  measures "d104" distance of L4.start L4.end
  measures "d105" distance of L5.start L5.end
  measures "d106" distance of L6.start L6.end
  measures "d107" diameter of A1
  measures "d108" diameter of A2
  measures "d109" diameter of A3
sketch "Sketch10" plane through (0, 0, 2.032) normal (0, 0, 1) x (-1, 0, 0)
  line L0 (-94.0435, -78.74) -> (-87.3125, -78.74)
  line L1 (-24.3205, -78.74) -> (-24.3205, -52.07)
  line L2 (-50.8635, -78.74) -> (-50.8635, -52.07)
  line L3 (-77.4065, -78.74) -> (-77.4065, -52.07)
  circle A0 centre (-24.3205, -52.07) radius 3.175
  circle A1 centre (-50.8635, -52.07) radius 3.175
  circle A2 centre (-77.4065, -52.07) radius 3.175
  line L4 (-6.604, -64.0804) -> (-6.604, -76.2)
  line L5 (-6.604, -76.2) -> (-1.905, -76.2)
  line L6 (-1.905, -76.2) -> (-1.905, 0)
  line L7 (-1.905, 0) -> (-99.695, 0)
  line L8 (-101.6, -76.2) -> (-92.7735, -76.2)
  line L9 (-92.7735, -76.2) -> (-92.7735, -77.47)
  line L10 (-92.7735, -77.47) -> (-94.0435, -77.47)
  line L11 (-94.0435, -77.47) -> (-94.0435, -78.74)
  line L12 (-87.3125, -78.74) -> (-87.3125, -77.47)
  line L13 (-87.3125, -77.47) -> (-88.5825, -77.47)
  line L14 (-88.5825, -77.47) -> (-88.5825, -76.2)
  line L15 (-88.5825, -76.2) -> (-86.233, -76.2)
  line L16 (-86.233, -76.2) -> (-95.123, -76.2)
  line L17 (-95.123, -76.2) -> (-95.123, -64.0804)
  line L18 (-95.123, -64.0804) -> (-86.233, -64.0804)
  line L19 (-86.233, -64.0804) -> (-86.233, -76.2)
  line L20 (-86.233, -76.2) -> (-79.502, -76.2)
  line L21 (-79.502, -76.2) -> (-79.502, -77.47)
  line L22 (-79.502, -77.47) -> (-80.772, -77.47)
  line L23 (-80.772, -77.47) -> (-80.772, -78.74)
  line L24 (-80.772, -78.74) -> (-74.0283, -78.74)
  line L25 (-74.0283, -78.74) -> (-74.0283, -77.47)
  line L26 (-74.0283, -77.47) -> (-75.2983, -77.47)
  line L27 (-75.2983, -77.47) -> (-75.2983, -76.2)
  line L28 (-75.2983, -76.2) -> (-74.295, -76.2)
  line L29 (-74.295, -76.2) -> (-69.215, -76.2)
  line L30 (-69.215, -76.2) -> (-68.58, -76.2)
  line L31 (-68.58, -76.2) -> (-68.58, -64.0804)
  line L32 (-68.58, -64.0804) -> (-59.69, -64.0804)
  line L33 (-59.69, -64.0804) -> (-59.69, -76.2)
  line L34 (-59.69, -76.2) -> (-66.2305, -76.2)
  line L35 (-66.2305, -76.2) -> (-66.2305, -77.47)
  line L36 (-66.2305, -77.47) -> (-67.5005, -77.47)
  line L37 (-67.5005, -77.47) -> (-67.5005, -78.74)
  line L38 (-67.5005, -78.74) -> (-60.7695, -78.74)
  line L39 (-60.7695, -78.74) -> (-60.7695, -77.47)
  line L40 (-60.7695, -77.47) -> (-62.0395, -77.47)
  line L41 (-62.0395, -77.47) -> (-62.0395, -76.2)
  line L42 (-62.0395, -76.2) -> (-59.055, -76.2)
  line L43 (-59.055, -76.2) -> (-52.959, -76.2)
  line L44 (-52.959, -76.2) -> (-52.959, -77.47)
  line L45 (-52.959, -77.47) -> (-54.229, -77.47)
  line L46 (-54.229, -77.47) -> (-54.229, -78.74)
  line L47 (-54.229, -78.74) -> (-47.498, -78.74)
  line L48 (-47.498, -78.74) -> (-47.498, -77.47)
  line L49 (-47.498, -77.47) -> (-48.768, -77.47)
  line L50 (-48.768, -77.47) -> (-48.768, -76.2)
  line L51 (-48.768, -76.2) -> (-39.6875, -76.2)
  line L52 (-39.6875, -76.2) -> (-39.6875, -77.47)
  line L53 (-39.6875, -77.47) -> (-40.9575, -77.47)
  line L54 (-40.9575, -77.47) -> (-40.9575, -78.74)
  line L55 (-40.9575, -78.74) -> (-34.2265, -78.74)
  line L56 (-34.2265, -78.74) -> (-34.2265, -77.47)
  line L57 (-34.2265, -77.47) -> (-35.4965, -77.47)
  line L58 (-35.4965, -77.47) -> (-35.4965, -76.2)
  line L59 (-35.4965, -76.2) -> (-27.432, -76.2)
  line L60 (-27.432, -76.2) -> (-26.416, -76.2)
  line L61 (-26.416, -76.2) -> (-26.416, -77.47)
  line L62 (-26.416, -77.47) -> (-27.686, -77.47)
  line L63 (-27.686, -77.47) -> (-27.686, -78.74)
  line L64 (-27.686, -78.74) -> (-20.955, -78.74)
  line L65 (-20.955, -78.74) -> (-20.955, -77.47)
  line L66 (-20.955, -77.47) -> (-22.225, -77.47)
  line L67 (-22.225, -77.47) -> (-22.225, -76.2)
  line L68 (-22.225, -76.2) -> (-21.209, -76.2)
  line L69 (-21.209, -76.2) -> (-15.494, -76.2)
  line L70 (-15.494, -76.2) -> (-15.494, -64.0804)
  line L71 (-15.494, -64.0804) -> (-6.604, -64.0804)
  line L72 (-75.5015, -64.0804) -> (-75.5015, -76.2)
  line L73 (-75.5015, -76.2) -> (-79.3115, -76.2)
  line L74 (-79.3115, -76.2) -> (-79.3115, -64.0804)
  line L75 (-79.3115, -64.0804) -> (-75.5015, -64.0804)
  line L76 (-22.4155, -64.0804) -> (-22.4155, -76.2)
  line L77 (-22.4155, -76.2) -> (-26.2255, -76.2)
  line L78 (-26.2255, -76.2) -> (-26.2255, -64.0804)
  line L79 (-26.2255, -64.0804) -> (-22.4155, -64.0804)
  line L80 (-48.9585, -64.0804) -> (-48.9585, -76.2)
  line L81 (-48.9585, -76.2) -> (-52.7685, -76.2)
  line L82 (-52.7685, -76.2) -> (-52.7685, -64.0804)
  line L83 (-52.7685, -64.0804) -> (-48.9585, -64.0804)
  line L84 (-33.147, -64.0804) -> (-33.147, -76.2)
  line L85 (-33.147, -76.2) -> (-42.037, -76.2)
  line L86 (-42.037, -76.2) -> (-42.037, -64.0804)
  line L87 (-42.037, -64.0804) -> (-33.147, -64.0804)
  line L88 (-99.695, 0) -> (-99.694, -76.2)
  line L89 (-99.694, -76.2) -> (-101.6, -76.2)
  dimension "d110" = 26.67
  dimension "d111" = 26.67
  dimension "d112" = 26.67
  dimension "d113" = 6.35
  dimension "d114" = 6.35
  dimension "d115" = 6.35
  constraint coincident L1.end A0.centre
  constraint coincident L2.end A1.centre
  constraint coincident L3.end A2.centre
  measures "d110" distance of L1.start L1.end
  measures "d111" distance of L2.start L2.end
  measures "d112" distance of L3.start L3.end
  measures "d113" diameter of A0
  measures "d114" diameter of A1
  measures "d115" diameter of A2
sketch "Sketch11" plane through (1.905, 0, 0) normal (1, 0, 0) x (0, 1, 0)
  circle A0 centre (66.04, 4.5174) radius 1.27
  line L0 (0, 2.032) -> (76.2, 2.032)
  line L1 (76.2, 2.032) -> (76.2, 12.192)
  line L2 (76.2, 12.192) -> (0, 12.192)
  line L3 (0, 12.192) -> (0, 2.032)
  line L4 (0, 2.032) -> (43, 2.032)
  line L5 (43, 2.032) -> (30.3, 2.032)
  line L6 (30.3, 2.032) -> (30.3, 6.032)
  line L7 (30.3, 6.032) -> (43, 6.032)
  line L8 (43, 6.032) -> (43, 2.032)
  line L9 (30.3, 6.032) -> (23.95, 6.032)
  line L10 (23.95, 6.032) -> (23.95, 2.0442)
  line L11 (23.95, 2.0442) -> (25.654, 2.032)
  dimension "d168" = 43
  dimension "d169" = 12.7
  dimension "d170" = 4
  dimension "d171" = 12.7
  dimension "d176" = 6.35
  dimension "d177" = 3.9878
  constraint coincident L0.start L3.end
  constraint perpendicular L3 L4
  constraint parallel L4 L5
  constraint perpendicular L4 L6
  constraint perpendicular L6 L7
  constraint perpendicular L6 L9
  constraint perpendicular L4 L10
  constraint coincident L4 L11.end
  measures "d168" distance of L0.start L4.end
  measures "d169" distance of L4.end L5.end
  measures "d170" distance of L5.end L6.end
  measures "d171" distance of L6.end L7.end
  measures "d176" distance of L6.end L9.end
  measures "d177" distance of L9.end L10.end
extrude "Extrude10" cut sketch "Sketch11" along normal blind 101.6 contours L0 L4 L6 L9 L10 L11 | L0 L4 L5 L6 L7 L8
extrude "Extrude11" cut sketch "Sketch11" against normal blind 7.62 contours L0 L4 L6 L9 L10 L11 | L0 L4 L5 L6 L7 L8
equation "d81 = 0.1 in - 0.025 in"
equation "d97 = 0.1 in - 0.025 in"
equation "d118 = ( 0.265 / 2 ) * 1 in"
equation "d119 = ( 0.265 / 2 ) * 1 in"
equation "d120 = ( 0.265 / 2 ) * 1 in"
equation "d121 = ( 0.265 / 2 ) * 1 in"
equation "d123 = ( 0.265 / 2 ) * 1 in"
equation "d124 = ( 0.265 / 2 ) * 1 in"
equation "d125 = ( 0.265 / 2 ) * 1 in"
equation "d126 = ( 0.265 / 2 ) * 1 in"
equation "d127 = ( 0.265 / 2 ) * 1 in"
equation "d129 = ( 0.265 / 2 ) * 1 in"
equation "d130 = ( 0.265 / 2 ) * 1 in"
equation "d131 = ( 0.265 / 2 ) * 1 in"
equation "d132 = ( 0.265 / 2 ) * 1 in"
